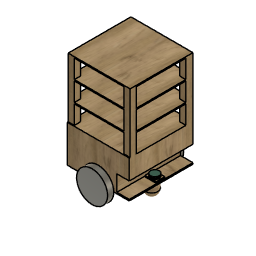
teddy v4 (Autodesk Fusion 360 design; units mm, degrees)
Autodesk Fusion 360 part; units mm, degrees
sketch "Sketch1" plane through (0, 0, 0) normal (0, 0, 1) x (1, 0, 0)
sketch "Sketch2" plane through (0, 0, 0) normal (0, 0, 1) x (1, 0, 0)
  line L0 (250, 256.8576) -> (-250, 256.8576)
  line L1 (-250, 256.8576) -> (-250, -256.8576)
  line L2 (-250, -256.8576) -> (250, -256.8576)
  line L3 (250, -256.8576) -> (250, 256.8576)
  line L4 (250, 256.8576) -> (-250, -256.8576) construction
  line L5 (-250, 256.8576) -> (250, -256.8576) construction
  dimension "d1" = 500
  constraint horizontal L0
  constraint perpendicular L0 L1
  constraint parallel L0 L2
  constraint parallel L1 L3
  constraint coincident L4 origin
  constraint coincident L5 origin
  measures "d1" distance of L1.end L2.end
extrude "Extrude1" add sketch "Sketch2" along normal blind 300 makes body 1
sketch "Sketch3" plane through (0, -256.8576, 0) normal (0, -1, 0) x (1, 0, 0)
  line L0 (-250, 0) -> (250, 0)
  line L1 (250, 0) -> (250, 300)
  line L2 (250, 300) -> (-250, 300)
  line L3 (-250, 300) -> (-250, 0)
  circle A0 centre (0, 125) radius 250
extrude "Extrude2" add sketch "Sketch3" along normal blind 75 separate body contours L0 L2 A0 | L0 A0 | L2 A0 makes body 2
mirror "Mirror1" about plane through (0, 0, 0) normal (0, 1, 0) of bodies 2 makes body 3
ref_plane "WorkPlane1" through (0, -309.803, -125) normal (0, 0, -1) x (-1, 0, 0)
sketch "Sketch4" plane through (0, 0, 0) normal (0, 0, -1) x (1, 0, 0)
  line L0 (250, -256.8576) -> (250, 256.8576)
  line L1 (250, 256.8576) -> (-250, 256.8576)
  line L2 (-250, 256.8576) -> (-250, -256.8576)
  line L3 (-250, -256.8576) -> (250, -256.8576)
  circle A0 centre (-175, 0) radius 50
  circle A1 centre (175, 0) radius 50
extrude "Extrude3" add sketch "Sketch4" along normal blind 125 contours A0 | A1 bodies 1
fillet "Fillet1" radius 50 1 faces at (-183.8876, -3.053, -125) on bodies 1
fillet "Fillet2" radius 50 1 faces at (169.821, 3.3706, -125) on bodies 1
move_body "Move1" bodies 1 2 3 to x (1, 0, 0) y (0, 1, 0) z (0, 0, 1) at (0, 0, 125)
sketch "Sketch5" plane through (-250, 0, 0) normal (-1, 0, 0) x (0, -1, 0)
  line L0 (-256.8576, 125) -> (256.8576, 125)
  line L1 (256.8576, 125) -> (256.8576, 425)
  line L2 (256.8576, 425) -> (-256.8576, 425)
  line L3 (-256.8576, 425) -> (-256.8576, 125)
  line L4 (147.3902, 135.6133) -> (-147.3902, 135.6133)
  line L5 (-147.3902, 135.6133) -> (-147.3902, 264.3867)
  line L6 (-147.3902, 264.3867) -> (147.3902, 264.3867)
  line L7 (147.3902, 264.3867) -> (147.3902, 135.6133)
  line L8 (147.3902, 135.6133) -> (-147.3902, 264.3867) construction
  line L9 (-147.3902, 135.6133) -> (147.3902, 264.3867) construction
  point P0 (0, 200)
  constraint horizontal L4
  constraint perpendicular L4 L5
  constraint parallel L4 L6
  constraint parallel L5 L7
  constraint coincident L8 P0
  constraint coincident L9 P0
extrude "Extrude4" cut sketch "Sketch5" against normal blind 100 contours L4 L5 L6 L7 bodies 1
sketch "Sketch6" plane through (0, 0, 135.6133) normal (0, 0, 1) x (-1, 0, 0)
  line L0 (250, -147.3902) -> (250, 147.3902)
  line L1 (250, 147.3902) -> (150, 147.3902)
  line L2 (150, 147.3902) -> (150, -147.3902)
  line L3 (150, -147.3902) -> (250, -147.3902)
  line L4 (245, 35) -> (155, 35)
  line L5 (155, 35) -> (155, -35)
  line L6 (155, -35) -> (245, -35)
  line L7 (245, -35) -> (245, 35)
  line L8 (245, 35) -> (155, -35) construction
  line L9 (155, 35) -> (245, -35) construction
  point P0 (200, 0)
  constraint horizontal L4
  constraint perpendicular L4 L5
  constraint parallel L4 L6
  constraint parallel L5 L7
  constraint coincident L8 P0
  constraint coincident L9 P0
extrude "Extrude5" add sketch "Sketch6" along normal blind 10 contours L4 L5 L6 L7 bodies 1
sketch "Sketch7" plane through (0, 0, 145.6133) normal (0, 0, 1) x (-1, 0, 0)
  line L0 (245, -35) -> (245, 35)
  line L1 (245, 35) -> (155, 35)
  line L2 (155, 35) -> (155, -35)
  line L3 (155, -35) -> (245, -35)
  circle A0 centre (200, 0) radius 35
  dimension "d19" = 70
  measures "d19" diameter of A0
extrude "Extrude6" add sketch "Sketch7" along normal blind 10 contours A0 bodies 1
extrude "Extrude7" add 1 faces at (-200.1229, -9.2059, 155.6133) along direction (0, 0, 1) blind 10 separate body on bodies 1 makes body 4
sketch "Sketch8" plane through (0, 0, 425) normal (0, 0, 1) x (-1, 0, 0)
  line L0 (-250, 256.8576) -> (-250, -256.8576)
  line L1 (-250, -256.8576) -> (250, -256.8576)
  line L2 (250, -256.8576) -> (250, 256.8576)
  line L3 (250, 256.8576) -> (-250, 256.8576)
  line L4 (-250, 200) -> (-200, 200)
  line L5 (-200, 200) -> (-200, 256.8576)
  line L6 (-200, 256.8576) -> (-250, 256.8576)
  line L7 (-250, 256.8576) -> (-250, 200)
  line L8 (-250, -200) -> (-200, -200)
  line L9 (-200, -200) -> (-200, -250)
  line L10 (-200, -250) -> (-250, -250)
  line L11 (-250, -250) -> (-250, -200)
  line L12 (200, -200) -> (250, -200)
  line L13 (250, -200) -> (250, -250)
  line L14 (250, -250) -> (200, -250)
  line L15 (200, -250) -> (200, -200)
  line L16 (200, 200) -> (250, 200)
  line L17 (250, 200) -> (250, 256.8576)
  line L18 (250, 256.8576) -> (200, 256.8576)
  line L19 (200, 256.8576) -> (200, 200)
  constraint perpendicular L4 L5
  constraint parallel L4 L6
  constraint parallel L5 L7
  constraint perpendicular L0 L4
  constraint coincident L0 L4.start
  constraint perpendicular L8 L9
  constraint parallel L8 L10
  constraint parallel L9 L11
  constraint perpendicular L0 L8
  constraint coincident L0 L8.start
  constraint perpendicular L12 L13
  constraint parallel L12 L14
  constraint parallel L13 L15
  constraint coincident L2 L12.end
  constraint perpendicular L2 L12
  constraint perpendicular L16 L17
  constraint parallel L16 L18
  constraint parallel L17 L19
  constraint coincident L2 L16.end
  constraint perpendicular L2 L16
extrude "Extrude8" add sketch "Sketch8" along normal blind 150 contours L0 L3 L4 L5 L6 L7 | L0 L8 L9 L10 L11 | L2 L3 L16 L17 L18 L19 | L2 L12 L13 L14 L15 bodies 1
sketch "Sketch9" plane through (0, 0, 575) normal (0, 0, 1) x (-1, 0, 0)
  line L0 (-250, 256.8576) -> (-250, 200)
  line L1 (-250, 200) -> (-200, 200)
  line L2 (-200, 200) -> (-200, 256.8576)
  line L3 (-200, 256.8576) -> (-250, 256.8576)
  line L4 (-250, 256.8576) -> (-250, -250)
  line L5 (-250, -250) -> (250, -250)
  line L6 (250, -250) -> (250, 256.8576)
  line L7 (250, 256.8576) -> (-250, 256.8576)
  constraint perpendicular L4 L5
  constraint parallel L4 L6
  constraint parallel L5 L7
  constraint perpendicular L3 L4
  constraint coincident L0.start L3.end
extrude "Extrude9" add sketch "Sketch9" along normal blind 10 bodies 1
sketch "Sketch10" plane through (0, 0, 585) normal (0, 0, 1) x (-1, 0, 0)
  line L0 (250, 256.8576) -> (-250, 256.8576)
  line L1 (-250, 256.8576) -> (-250, -250)
  line L2 (-250, -250) -> (250, -250)
  line L3 (250, -250) -> (250, 256.8576)
  line L4 (-200, 200) -> (-250, 200)
  line L5 (-250, 200) -> (-250, 256.8576)
  line L6 (-250, 256.8576) -> (-200, 256.8576)
  line L7 (-200, 256.8576) -> (-200, 200)
  line L8 (250, 200) -> (200, 200)
  line L9 (200, 200) -> (200, 256.8576)
  line L10 (200, 256.8576) -> (250, 256.8576)
  line L11 (250, 256.8576) -> (250, 200)
  line L12 (250, -200) -> (200, -200)
  line L13 (200, -200) -> (200, -250)
  line L14 (200, -250) -> (250, -250)
  line L15 (250, -250) -> (250, -200)
  line L16 (-200, -200) -> (-250, -200)
  line L17 (-250, -200) -> (-250, -250)
  line L18 (-250, -250) -> (-200, -250)
  line L19 (-200, -250) -> (-200, -200)
  constraint perpendicular L4 L5
  constraint parallel L4 L6
  constraint parallel L5 L7
  constraint coincident L1 L4.end
  constraint perpendicular L1 L4
  constraint perpendicular L8 L9
  constraint parallel L8 L10
  constraint parallel L9 L11
  constraint perpendicular L3 L8
  constraint coincident L3 L8.start
  constraint perpendicular L12 L13
  constraint parallel L12 L14
  constraint parallel L13 L15
  constraint perpendicular L3 L12
  constraint coincident L3 L12.start
  constraint perpendicular L16 L17
  constraint parallel L16 L18
  constraint parallel L17 L19
  constraint coincident L1 L16.end
  constraint perpendicular L1 L16
extrude "Extrude10" add sketch "Sketch10" along normal blind 150 contours L0 L3 L8 L9 L10 L11 | L0 L1 L4 L5 L6 L7 | L2 L3 L12 L13 L14 L15 | L1 L2 L16 L17 L18 L19 bodies 1
sketch "Sketch11" plane through (0, 0, 735) normal (0, 0, 1) x (-1, 0, 0)
  line L0 (-200, 256.8576) -> (-250, 256.8576)
  line L1 (-250, 256.8576) -> (-250, 200)
  line L2 (-250, 200) -> (-200, 200)
  line L3 (-200, 200) -> (-200, 256.8576)
  line L4 (-250, 256.8576) -> (-250, -250)
  line L5 (-250, -250) -> (250, -250)
  line L6 (250, -250) -> (250, 256.8576)
  line L7 (250, 256.8576) -> (-250, 256.8576)
  constraint perpendicular L4 L5
  constraint parallel L4 L6
  constraint parallel L5 L7
  constraint perpendicular L2 L4
  constraint coincident L0.end L1.start
extrude "Extrude11" add sketch "Sketch11" along normal blind 10 bodies 1
sketch "Sketch12" plane through (0, 0, 745) normal (0, 0, 1) x (-1, 0, 0)
  line L0 (250, 256.8576) -> (-250, 256.8576)
  line L1 (-250, 256.8576) -> (-250, -250)
  line L2 (-250, -250) -> (250, -250)
  line L3 (250, -250) -> (250, 256.8576)
  line L4 (-200, 200) -> (-250, 200)
  line L5 (-250, 200) -> (-250, 256.8576)
  line L6 (-250, 256.8576) -> (-200, 256.8576)
  line L7 (-200, 256.8576) -> (-200, 200)
  line L8 (250, 200) -> (200, 200)
  line L9 (200, 200) -> (200, 256.8576)
  line L10 (200, 256.8576) -> (250, 256.8576)
  line L11 (250, 256.8576) -> (250, 200)
  line L12 (-200, -200) -> (-250, -200)
  line L13 (-250, -200) -> (-250, -250)
  line L14 (-250, -250) -> (-200, -250)
  line L15 (-200, -250) -> (-200, -200)
  line L16 (250, -200) -> (200, -200)
  line L17 (200, -200) -> (200, -250)
  line L18 (200, -250) -> (250, -250)
  line L19 (250, -250) -> (250, -200)
  constraint perpendicular L4 L5
  constraint parallel L4 L6
  constraint parallel L5 L7
  constraint coincident L1 L4.end
  constraint perpendicular L1 L4
  constraint perpendicular L8 L9
  constraint parallel L8 L10
  constraint parallel L9 L11
  constraint perpendicular L3 L8
  constraint coincident L3 L8.start
  constraint perpendicular L12 L13
  constraint parallel L12 L14
  constraint parallel L13 L15
  constraint coincident L1 L12.end
  constraint perpendicular L1 L12
  constraint perpendicular L16 L17
  constraint parallel L16 L18
  constraint parallel L17 L19
  constraint perpendicular L3 L16
  constraint coincident L3 L16.start
extrude "Extrude12" add sketch "Sketch12" along normal blind 150 contours L0 L3 L8 L9 L10 L11 | L0 L1 L4 L5 L6 L7 | L2 L3 L16 L17 L18 L19 | L1 L2 L12 L13 L14 L15 bodies 1
sketch "Sketch13" plane through (0, 0, 895) normal (0, 0, 1) x (-1, 0, 0)
  line L0 (-200, 256.8576) -> (-250, 256.8576)
  line L1 (-250, 256.8576) -> (-250, 200)
  line L2 (-250, 200) -> (-200, 200)
  line L3 (-200, 200) -> (-200, 256.8576)
  line L4 (-250, 256.8576) -> (-250, -250)
  line L5 (-250, -250) -> (250, -250)
  line L6 (250, -250) -> (250, 256.8576)
  line L7 (250, 256.8576) -> (-250, 256.8576)
  constraint perpendicular L4 L5
  constraint parallel L4 L6
  constraint parallel L5 L7
  constraint perpendicular L0 L4
  constraint coincident L0.end L1.start
extrude "Extrude13" add sketch "Sketch13" along normal blind 10 bodies 1
delete_body "RemoveBody1" bodies 3
sketch "Sketch14" plane through (0, 256.8576, 0) normal (0, 1, 0) x (-1, 0, 0)
  line L0 (-250, 125) -> (250, 125)
  line L1 (250, 125) -> (250, 425)
  line L2 (250, 425) -> (-250, 425)
  line L3 (-250, 425) -> (-250, 125)
  circle A0 centre (0, 275) radius 275
  constraint coincident origin A0
extrude "Extrude14" add sketch "Sketch14" along normal blind 50 separate body contours L0 L1 L2 L3 A0 | L0 A0 | L3 A0 | L1 A0 | L2 A0 makes body 5
delete_body "RemoveBody2" bodies 2
mirror "Mirror2" about plane through (0, 0, 0) normal (0, 1, 0) of bodies 5 makes body 6
move_body "Move2" bodies 6 5 1 4 to x (-1, 0, 0) y (0, -1, 0) z (0, 0, 1) at (-550, -613.7152, 0)
move_body "Move3" bodies 4 1 5 6 to x (1, 0, 0) y (0, 1, 0) z (0, 0, 1) at (550, 600, 0)
move_body "Move4" bodies 4 6 1 5 to x (1, 0, 0) y (0, 1, 0) z (0, 0, 1) at (0, 15, 0)
delete_body "RemoveBody3" bodies 6
sketch "Sketch15" plane through (0, 258.1424, 0) normal (0, 1, 0) x (-1, 0, 0)
  line L0 (-250, 905) -> (-250, 125)
  line L1 (-250, 125) -> (250, 125)
  line L2 (250, 125) -> (250, 905)
  line L3 (250, 905) -> (-250, 905)
  line L4 (-200, 895) -> (200, 895)
  line L5 (200, 895) -> (200, 745)
  line L6 (200, 745) -> (-200, 745)
  line L7 (-200, 745) -> (-200, 895)
  line L8 (-200, 735) -> (200, 735)
  line L9 (200, 735) -> (200, 585)
  line L10 (200, 585) -> (-200, 585)
  line L11 (-200, 585) -> (-200, 735)
  line L12 (-200, 575) -> (200, 575)
  line L13 (200, 575) -> (200, 425)
  line L14 (200, 425) -> (-200, 425)
  line L15 (-200, 425) -> (-200, 575)
  circle A0 centre (0, 125) radius 125
  constraint midpoint L1 A0.centre
  constraint coincident origin A0
extrude "Extrude15" add sketch "Sketch15" along normal blind 50 separate body contours L1 A0 | L1 A0 makes body 7
delete_body "RemoveBody4" bodies 5
sketch "Sketch16" plane through (0, -255.5729, 0) normal (0, -1, 0) x (1, 0, 0)
  line L0 (-250, 125) -> (250, 125)
  line L1 (250, 125) -> (250, 425)
  line L2 (250, 425) -> (-250, 425)
  line L3 (-250, 425) -> (-250, 125)
  circle A0 centre (0, 125) radius 125
  constraint midpoint L0 A0.centre
  constraint coincident origin A0
extrude "Extrude16" add sketch "Sketch16" along normal blind 50 separate body contours L0 A0 | L0 A0 makes body 8
copy_body "Body->Comp1" bodies 1 removing the originals makes body 9 in component "base_link"
copy_body "Body->Comp2" bodies 4 removing the originals makes body 10 in component "lidar"
copy_body "Body->Comp3" bodies 7 removing the originals makes body 11 in component "right_wheel"
copy_body "Body->Comp4" bodies 8 removing the originals makes body 12 in component "left_wheel"
sketch "Sketch17" plane through (250, 0, 0) normal (1, 0, 0) x (0, 1, 0)
  line L0 (201.2848, 895) -> (201.2848, 745)
  line L1 (201.2848, 745) -> (-198.7152, 745)
  line L2 (-198.7152, 745) -> (-198.7152, 895)
  line L3 (-198.7152, 895) -> (201.2848, 895)
  line L4 (201.2848, 735) -> (201.2848, 585)
  line L5 (201.2848, 585) -> (-198.7152, 585)
  line L6 (-198.7152, 585) -> (-198.7152, 735)
  line L7 (-198.7152, 735) -> (201.2848, 735)
  line L8 (258.1424, 125) -> (258.1424, 905)
  line L9 (258.1424, 905) -> (-248.7152, 905)
  line L10 (-248.7152, 905) -> (-248.7152, 425)
  line L11 (-248.7152, 425) -> (-255.5729, 425)
  line L12 (-255.5729, 425) -> (-255.5729, 125)
  line L13 (-255.5729, 125) -> (258.1424, 125)
  line L14 (-146.1054, 135.6133) -> (-146.1054, 264.3867)
  line L15 (-146.1054, 264.3867) -> (148.675, 264.3867)
  line L16 (148.675, 264.3867) -> (148.675, 135.6133)
  line L17 (148.675, 135.6133) -> (-146.1054, 135.6133)
  line L18 (-198.7152, 575) -> (201.2848, 575)
  line L19 (201.2848, 575) -> (201.2848, 425)
  line L20 (201.2848, 425) -> (-198.7152, 425)
  line L21 (-198.7152, 425) -> (-198.7152, 575)
  line L22 (258.1424, 135.6133) -> (-258.1424, 135.6133)
  line L23 (-258.1424, 135.6133) -> (-258.1424, 264.3867)
  line L24 (-258.1424, 264.3867) -> (258.1424, 264.3867)
  line L25 (258.1424, 264.3867) -> (258.1424, 135.6133)
  line L26 (258.1424, 135.6133) -> (-258.1424, 264.3867) construction
  line L27 (-258.1424, 135.6133) -> (258.1424, 264.3867) construction
  point P0 (0, 200)
  constraint horizontal L22
  constraint perpendicular L22 L23
  constraint parallel L22 L24
  constraint parallel L23 L25
  constraint coincident L26 P0
  constraint coincident L27 P0
  constraint coincident L8 L22.start
extrude "Extrude1'" cut sketch "Sketch17" against normal blind 100 contours L8 L16 L22 L24 L25 | L12 L14 L22 L24 bodies 9 in component "base_link"
component "base_link" placed x (1, 0, 0) y (0, 1, 0) z (0, 0, 1) at (0, 0, 0)
component "lidar" placed x (1, 0, 0) y (0, 1, 0) z (0, 0, 1) at (0, 0, 0)
component "right_wheel" placed x (1, 0, 0) y (0, 1, 0) z (0, 0, 1) at (0, 0, 0)
component "left_wheel" placed x (1, 0, 0) y (0, 1, 0) z (0, 0, 1) at (0, 0, 0)
named bodies: "base_link", "right_wheel", "left_wheel", "lidar"
